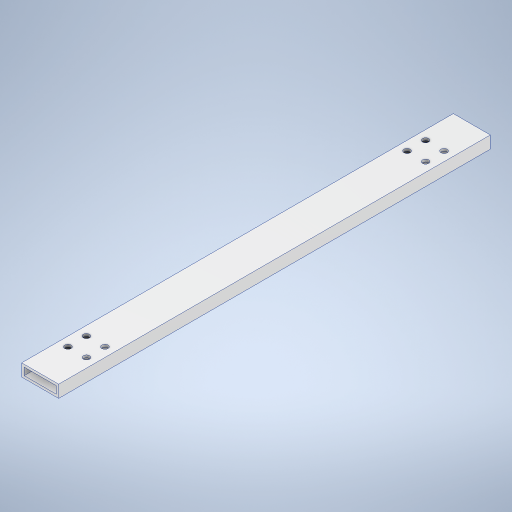
# Autodesk Inventor part: long_frame
Saved by Autodesk Inventor 2023 (Build 270158000, 158)
## iProperties
Created: 2023-04-12
Part Number: long_frame
Material: Aluminum 6061
Document SubType Name: Modeling
Designer: LAB-505
Density: 2.7 g/cm^3
Appearance: Aluminum - Flat
Mass: 134.384 g
Surface Area: 505.623 cm^2
Volume: 49.7717 cm^3
Author: LAB-505
Autodesk Inventor part; units mm, degrees
ref_plane "YZ Plane" through (0, 0, 0) normal (1, 0, 0) x (0, 1, 0)
ref_plane "XZ Plane" through (0, 0, 0) normal (0, 1, 0) x (-1, 0, 0)
ref_plane "XY Plane" through (0, 0, 0) normal (0, 0, 1) x (1, 0, 0)
sketch "Sketch2" plane through (0, 0, 0) normal (0, 0, 1) x (1, 0, 0)
  line L0 (0, 0) -> (30, 0)
  line L1 (30, 0) -> (30, 10)
  line L2 (30, 10) -> (0, 10)
  line L3 (0, 10) -> (0, 0)
  line L4 (2.0014, 2) -> (28.0014, 2)
  line L5 (28.0014, 2) -> (28.0014, 8)
  line L6 (28.0014, 8) -> (2.0014, 8)
  line L7 (2.0014, 8) -> (2.0014, 2)
  dimension "d0" = 30
  dimension "d1" = 10
  dimension "d2" = 26
  dimension "d3" = 6
  constraints: 16 end point, 4 parallel, 2 horizontal, 2 perpendicular
  measures "d0" distance of L2.end L1.end
  measures "d1" distance of L1.end L0.end
  measures "d2" distance of L6.end L5.end
  measures "d3" distance of L5.end L4.end
extrude "Extrusion1" add sketch "Sketch2" along normal blind 350
sketch "Sketch3" plane through (0, 10, 0) normal (0, 1, 0) x (1, 0, 0)
  circle A0 centre (7.5, -30) radius 2.5
  circle A1 centre (22.5, -30) radius 2.5
  circle A2 centre (7.5, -45) radius 2.5
  circle A3 centre (22.5, -45) radius 2.5
  circle A4 centre (7.5, -320) radius 2.5
  circle A5 centre (22.5, -320) radius 2.5
  circle A6 centre (7.5, -305) radius 2.5
  circle A7 centre (22.5, -305) radius 2.5
  point P0 (0, 0)
  dimension "d6" = 5
  dimension "d7" = 5
  dimension "d8" = 5
  dimension "d9" = 5
  dimension "d10" = 5
  dimension "d11" = 5
  dimension "d12" = 5
  dimension "d13" = 5
  constraints: 8 centre point
  measures "d6" diameter of A0
  measures "d7" diameter of A1
  measures "d8" diameter of A2
  measures "d9" diameter of A3
  measures "d10" diameter of A4
  measures "d11" diameter of A5
  measures "d12" diameter of A6
  measures "d13" diameter of A7
extrude "Extrusion2" cut sketch "Sketch3" against normal blind 169.1125
body "Solid1"
